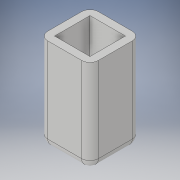
# Autodesk Inventor part: 1in_2020_Endcap
Saved by Autodesk Inventor 2019.4 (Build 234330000, 330)
## iProperties
Created: 2020-03-13
Part Number: 1in_2020_Endcap
Material: Generic
Document SubType Name: Modeling
Designer: Jorian Bruslind
Density: 1 g/cm^3
Appearance: Default
Author: Jorian Bruslind
Autodesk Inventor part; units mm, degrees
ref_plane "YZ Plane" through (0, 0, 0) normal (1, 0, 0) x (0, 1, 0)
ref_plane "XZ Plane" through (0, 0, 0) normal (0, 1, 0) x (-1, 0, 0)
ref_plane "XY Plane" through (0, 0, 0) normal (0, 0, 1) x (1, 0, 0)
sketch "Sketch1" plane through (0, 0, 0) normal (0, 1, 0) x (-1, 0, 0)
  line L0 (0, 0) -> (30, 0)
  line L1 (30, 0) -> (30, -30)
  line L2 (30, -30) -> (0, -30)
  line L3 (0, -30) -> (0, 0)
  dimension "d0" = 30
  dimension "d1" = 30
  constraints: 8 end point, 2 parallel, 1 horizontal, 1 perpendicular
  measures "d0" distance of L1.end L2.end
  measures "d1" distance of L0.end L1.end
extrude "Extrusion1" add sketch "Sketch1" along normal blind 55.4
sketch "Sketch2" plane through (0, 55.4, 0) normal (0, 1, 0) x (1, 0, 0)
  line L0 (0, 0) -> (0, 30) projected
  line L1 (0, 0) -> (0, 4.5)
  line L2 (0, 4.5) -> (-4.5, 4.5)
  line L3 (-4.5, 4.5) -> (-25.5, 4.5)
  line L4 (-25.5, 4.5) -> (-25.5, 25.5)
  line L5 (-25.5, 25.5) -> (-4.5, 25.5)
  line L6 (-4.5, 25.5) -> (-4.5, 4.5)
  dimension "d4" = 4.5
  dimension "d5" = 4.5
  dimension "d6" = 21
  dimension "d7" = 21
  constraints: 12 end point, 2 parallel, 2 perpendicular, 1 horizontal, 1 point on line
  measures "d4" distance of L0.start L1.end
  measures "d5" distance of L1.end L2.end
  measures "d6" distance of L4.end L5.end
  measures "d7" distance of L3.end L4.end
extrude "Extrusion2" cut sketch "Sketch2" against normal blind 30
sketch "Sketch3" plane through (0, 0, 0) normal (0, -1, 0) x (1, 0, 0)
  line L0 (0, 0) -> (-15, 0)
  line L1 (0, 0) -> (-30, 0) projected
  line L2 (-15, 0) -> (-15, -15)
  circle A0 centre (-15, -15) radius 2
  dimension "d10" = 15
  dimension "d11" = 4
  constraints: 4 end point, 1 centre point, 1 coincident, 1 midpoint, 1 perpendicular
  measures "d10" distance of L0.end L2.end
  measures "d11" diameter of A0
extrude "Extrusion3" cut sketch "Sketch3" against normal blind 5
fillet "Fillet1" radius 5 4 edges at (0, 0, -15) (-15, 0, 0) (-15, 0, -30) (-30, 0, -15)
fillet "Fillet2" radius 5 8 edges at (-1.4645, 1.4645, -28.5355) (0, 30.2, -30) (-1.4645, 1.4645, -1.4645) (0, 30.2, 0) (-28.5355, 1.4645, -28.5355) (-30, 30.2, -30) (-28.5355, 1.4645, -1.4645) (-30, 30.2, 0)
body "Solid1"
